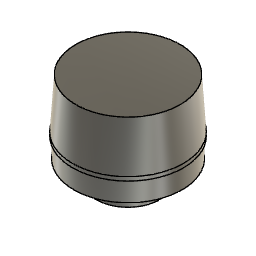
Knob_v1_model_for_checking_enclosure_design (Autodesk Fusion 360 design; units mm, degrees)
Autodesk Fusion 360 part; units mm, degrees
sketch "スケッチ1" plane through (0, 0, 0) normal (0, 0, 1) x (1, 0, 0)
  circle A0 centre (0, 0) radius 14.25
  dimension "d1" = 28.5
  constraint coincident A0.centre origin
  measures "d1" diameter of A0
extrude "押し出し1" add sketch "スケッチ1" along normal blind 5.2
sketch "スケッチ2" plane through (0, 0, 5.2) normal (0, 0, 1) x (-1, 0, 0)
  circle A0 centre (0, 0) radius 14.25
  circle A1 centre (0, 0) radius 14.6
  dimension "d4" = 29.2
  constraint concentric A0 A1
  measures "d4" diameter of A1
extrude "押し出し2" add sketch "スケッチ2" along normal blind 1 contours A0 | A1
sketch "スケッチ3" plane through (0, 0, 6.2) normal (0, 0, 1) x (-1, 0, 0)
  circle A0 centre (0, 0) radius 14.6
  circle A1 through (13.75, 0, 13) (-6.875, 11.9078, 13) (-6.875, -11.9078, 13)
  dimension "d8" = 27.5
loft "ロフト1" add profiles "スケッチ3", "スケッチ3" section 1 section 2 contours A1 in plane through (0, 0, 19.2) normal (0, 0, 1)
sketch "スケッチ4" plane through (0, 0, 0) normal (0, 0, -1) x (1, 0, 0)
  circle A0 centre (0, 0) radius 14.25
  circle A1 centre (0, 0) radius 8.35
  dimension "d9" = 16.7
  constraint concentric A0 A1
  measures "d9" diameter of A1
extrude "押し出し3" add sketch "スケッチ4" along normal blind 5.2 contours A1
sketch "スケッチ5" plane through (0, 0, -5.2) normal (0, 0, -1) x (1, 0, 0)
  circle A0 centre (0, 0) radius 8.35
  circle A1 centre (0, 0) radius 3.5
  dimension "d12" = 7
  constraint concentric A0 A1
  measures "d12" diameter of A1
extrude "押し出し4" cut sketch "スケッチ5" against normal blind 5.2 contours A1
sketch "スケッチ6" plane through (0, 0, 0) normal (0, 0, -1) x (1, 0, 0)
  circle A0 centre (0, 0) radius 3.5
  circle A1 centre (0, 0) radius 3
  line L0 (-1.5, 3.1623) -> (-1.5, -3.1623)
  dimension "d15" = 6
  dimension "d16" = 1.5
  constraint coincident A0.centre A1.centre
  constraint coincident A0 L0.start
  constraint coincident A0 L0.end
  constraint vertical L0
  measures "d15" diameter of A1
  measures "d16" distance of A0.centre L0
extrude "押し出し5" cut sketch "スケッチ6" against normal blind 15.6 contours A1 L0 picked at (1.1235, 0.0842)
equation "d17 = -20.8 mm + 5.2 mm"
